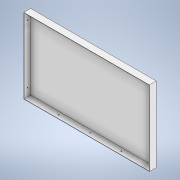
# Autodesk Inventor part: Tapa_superior_derecha
Saved by Autodesk Inventor 2021 (Build 250183000, 183)
## iProperties
Created: 2021-04-15
Part Number: Tapa_superior_derecha
Material: Acero AISI 1006 85 LC
Document SubType Name: Modeling
Designer: Admin
Density: 7.872 g/cm^3
Appearance: Blanco
Mass: 809.634 g
Surface Area: 2272.26 cm^2
Volume: 102.85 cm^3
Author: Admin
Autodesk Inventor part; units mm, degrees
ref_plane "YZ Plane" through (0, 0, 0) normal (1, 0, 0) x (0, 1, 0)
ref_plane "XZ Plane" through (0, 0, 0) normal (0, 1, 0) x (-1, 0, 0)
ref_plane "XY Plane" through (0, 0, 0) normal (0, 0, 1) x (1, 0, 0)
sketch "Boceto1" plane through (0, 0, 0) normal (0, 0, 1) x (1, 0, 0)
  line L0 (0, 0) -> (385, 0)
  line L1 (385, 0) -> (385, 230)
  line L2 (385, 230) -> (0, 230)
  line L3 (0, 230) -> (0, 0)
  dimension "d0" = 385
  dimension "d1" = 230
  constraints: 8 end point, 2 parallel, 1 horizontal, 1 perpendicular
  measures "d0" distance of L2.end L1.end
  measures "d1" distance of L1.end L0.end
extrude "Extrusión1" add sketch "Boceto1" along normal blind 0.91
sketch "Boceto2" plane through (0, 0, 0.91) normal (0, 0, 1) x (1, 0, 0)
  line L0 (385, 230) -> (0, 230) projected
  line L1 (0, 0) -> (0.76, 0)
  line L2 (0.91, 0.91) -> (0.91, 229.09)
  line L3 (0.91, 230) -> (0, 230)
  line L4 (0, 230) -> (0, 0)
  line L5 (0, 230) -> (0, 0) projected
  line L6 (385, 0) -> (385, 230) projected
  line L7 (0, 0) -> (385, 0)
  line L8 (385, 0) -> (385, 0.91)
  line L9 (384.09, 0.91) -> (0.91, 0.91)
  line L10 (0, 0.76) -> (0, 0)
  line L11 (0, 0) -> (385, 0) projected
  line L12 (385, 0) -> (384.24, 0)
  line L13 (384.09, 0.91) -> (384.09, 229.09)
  line L14 (384.09, 230) -> (385, 230)
  line L15 (385, 230) -> (385, 0)
  line L16 (385, 230) -> (0, 230)
  line L17 (0, 230) -> (0, 229.09)
  line L18 (0.91, 229.09) -> (384.09, 229.09)
  line L19 (385, 229.24) -> (385, 230)
  dimension "d36" = 0.91
  dimension "d37" = 0.91
  dimension "d38" = 0.91
  dimension "d39" = 0.91
  constraints: 32 end point, 8 parallel, 4 horizontal, 4 perpendicular, 4 point on line
  measures "d36" distance between parallel lines of L7 L9
  measures "d37" distance between parallel lines of L6 L13
  measures "d38" distance between parallel lines of L5 L2
  measures "d39" distance between parallel lines of L0 L18
extrude "Extrusión2" add sketch "Boceto2" along normal blind 20
sketch "Boceto3" plane through (0, 0, 0) normal (0, 0, -1) x (-1, 0, 0)
  line L0 (-384.09, 0.91) -> (-384.09, 229.09) projected
  line L1 (-0.91, 0.91) -> (-384.09, 0.91) projected
  line L2 (-365.39, 0.91) -> (-351.39, 0.91) construction
  circle A0 centre (-365.24, 14.76) radius 1
  line L3 (-385, 230) -> (-366, 230)
  line L4 (-385, 230) -> (0, 230) projected
  line L5 (-366, 230) -> (-366, 216)
  circle A1 centre (-366, 216) radius 1.5875
  line L6 (-366, 216) -> (-108, 216)
  circle A2 centre (-108, 216) radius 1.5875
  point P0 (0, 0)
  dimension "d14" = 19
  dimension "d15" = 14
  dimension "d16" = 90
  dimension "d17" = 3.175
  dimension "d18" = 258
  dimension "d19" = 3.175
  constraints: 8 end point, 3 centre point, 2 coincident, 2 horizontal, 2 point on line, 1 perpendicular
  measures "d14" distance of L3.start L3.end
  measures "d15" distance of L3.end L5.end
  measures "d16" angle of L3 L5
  measures "d17" diameter of A1
  measures "d18" distance of L6.start L6.end
  measures "d19" diameter of A2
extrude "Extrusión3" cut sketch "Boceto3" against normal through all contours A1 L6 L5 | L5 L6 A1 | A2
sketch "Boceto4" plane through (0, 0, 0) normal (0, -1, 0) x (1, 0, 0)
  line L0 (0, 0) -> (0, 20.91) construction
  line L1 (0, 10.455) -> (385, 10.455) construction
  line L2 (385, 0) -> (385, 20.91) construction
  line L3 (0, 10.455) -> (96.25, 10.455) construction
  line L4 (96.25, 10.455) -> (192.5, 10.455) construction
  line L5 (192.5, 10.455) -> (288.75, 10.455) construction
  circle A0 centre (96.25, 10.455) radius 1.5875
  circle A1 centre (192.5, 10.455) radius 1.5875
  circle A2 centre (288.75, 10.455) radius 1.5875
  dimension "d22" = 96.25
  dimension "d23" = 96.25
  dimension "d24" = 96.25
  dimension "d25" = 3.175
  dimension "d26" = 3.175
  dimension "d27" = 3.175
  constraints: 8 end point, 3 centre point, 3 coincident, 3 midpoint, 2 point on line
  measures "d22" distance of L1.start L3.end
  measures "d23" distance of L3.end L4.end
  measures "d24" distance of L4.end L5.end
  measures "d25" diameter of A0
  measures "d26" diameter of A1
  measures "d27" diameter of A2
ref_plane "Plano de trabajo1" through (1.52, 1.52, 0.76) normal (0, 1, 0) x (0, 0, 1)
extrude "Extrusión4" cut sketch "Boceto4" against normal up to surface (1.52 mm away)
sketch "Boceto5" plane through (0, 0, 0) normal (-1, 0, 0) x (0, 0, 1)
  line L0 (0, 0) -> (20.91, 0) construction
  line L1 (10.455, 0) -> (10.455, 230) construction
  line L2 (0, 230) -> (20.91, 230) construction
  line L3 (10.455, 0) -> (10.455, 25.4) construction
  line L4 (10.455, 230) -> (10.455, 204.6) construction
  circle A0 centre (10.455, 25.4) radius 1.5875
  circle A1 centre (10.455, 204.6) radius 1.5875
  dimension "d30" = 25.4
  dimension "d31" = 25.4
  dimension "d32" = 3.175
  dimension "d33" = 3.175
  constraints: 6 end point, 2 centre point, 2 coincident, 2 midpoint, 2 point on line
  measures "d30" distance of L1.start L3.end
  measures "d31" distance of L1.end L4.end
  measures "d32" diameter of A0
  measures "d33" diameter of A1
ref_plane "Plano de trabajo2" through (1.52, 1.52, 0.76) normal (1, 0, 0) x (0, 1, 0)
extrude "Extrusión5" cut sketch "Boceto5" against normal up to surface (1.52 mm away)
